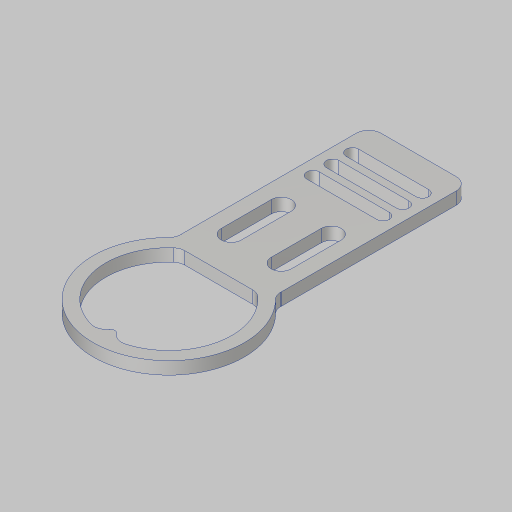
# Autodesk Inventor part: EL2-C-006
Saved by Autodesk Inventor 2023.5 (Build 275446000, 446)
## iProperties
Created: 2025-01-21
Part Number: EL2-C-006
Material: Aluminum 6061
Document SubType Name: Modeling
Designer: slick
Density: 2.7 g/cm^3
Appearance: Aluminum - Flat
Author: slick
Autodesk Inventor part; units mm, degrees
ref_plane "YZ Plane" through (0, 0, 0) normal (1, 0, 0) x (0, 1, 0)
ref_plane "XZ Plane" through (0, 0, 0) normal (0, 1, 0) x (-1, 0, 0)
ref_plane "XY Plane" through (0, 0, 0) normal (0, 0, 1) x (1, 0, 0)
sketch "Sketch1" plane through (0, 0, 0) normal (0, 1, 0) x (-1, 0, 0)
  line L0 (8.89, 0) -> (-8.89, 0) construction
  line L1 (8.89, 1.5875) -> (-8.89, 1.5875)
  line L2 (-8.89, -1.5875) -> (8.89, -1.5875)
  arc A0 (8.89, -1.5875) -> (8.89, 1.5875) centre (8.89, 0) ccw
  arc A1 (-8.89, 1.5875) -> (-8.89, -1.5875) centre (-8.89, 0) ccw
  line L3 (8.89, -5.0038) -> (-8.89, -5.0038) construction
  line L4 (8.89, -3.4163) -> (-8.89, -3.4163)
  line L5 (-8.89, -6.5913) -> (8.89, -6.5913)
  arc A2 (8.89, -6.5913) -> (8.89, -3.4163) centre (8.89, -5.0038) ccw
  arc A3 (-8.89, -3.4163) -> (-8.89, -6.5913) centre (-8.89, -5.0038) ccw
  line L6 (8.89, -10.0076) -> (-8.89, -10.0076) construction
  line L7 (8.89, -8.4201) -> (-8.89, -8.4201)
  line L8 (-8.89, -11.5951) -> (8.89, -11.5951)
  arc A4 (8.89, -11.5951) -> (8.89, -8.4201) centre (8.89, -10.0076) ccw
  arc A5 (-8.89, -8.4201) -> (-8.89, -11.5951) centre (-8.89, -10.0076) ccw
  line L9 (12.7, 32.8549) -> (-12.7, 32.8549)
  line L10 (-12.7, 32.8549) -> (-12.7, -17.9451)
  line L11 (-12.7, -17.9451) -> (12.7, -17.9451)
  line L12 (12.7, -17.9451) -> (12.7, 32.8549)
  line L13 (6.35, 26.5049) -> (-6.35, 26.5049) construction
  point P0 (0, 0)
  point P1 (0, -5.0038)
  point P2 (0, -10.0076)
  point P3 (10.4775, -5.0038)
  point P4 (10.4775, 0)
  point P5 (10.4775, -10.0076)
  point P6 (0, -17.9451)
  point P7 (0, -11.5951)
  point P8 (0, 26.5049)
  point P9 (0, 32.8549)
  dimension "d1" = 17.78
  dimension "d3" = 3.175
  dimension "d4" = 5.0038
  dimension "d5" = 5.0038
  dimension "d8" = 25.4
  dimension "d9" = 50.8
  dimension "d10" = 6.35
  dimension "d11" = 12.7
  dimension "d12" = 6.35
  constraints: 34 end point, 15 point on circle, 12 tangent, 9 parallel, 7 midpoint, 6 centre point, 4 vertical alignment, 3 horizontal, 2 equal radius, 1 horizontal alignment, 1 perpendicular
  measures "d1" distance of L1.start L1.end
  measures "d3" distance between parallel lines of L2 L1
  measures "d4" distance of point (10.477, -5.004) point (10.477, 0)
  measures "d5" distance of point (10.477, -10.008) point (10.477, -5.004)
  measures "d8" distance of L10.end L11.end
  measures "d9" distance of L11.end L9.start
  measures "d10" distance of point (0, -11.595) point (0, -17.945)
  measures "d11" distance of L13.start L13.end
  measures "d12" distance from line of L9 L13.start
extrude "Extrusion1" add sketch "Sketch1" along normal blind 3.175
fillet "Fillet1" radius 3.175 4 edges at (-12.7, 1.5875, -17.9451) (12.7, 1.5875, -17.9451) (12.7, 1.5875, 32.8549) (-12.7, 1.5875, 32.8549)
sketch "Sketch2" plane through (0, 3.175, 0) normal (0, 1, 0) x (1, 0, 0)
  line L0 (-6.35, -10.6299) -> (-6.35, -23.3299) construction
  line L1 (-8.9027, -10.6299) -> (-8.9027, -23.3299)
  line L2 (-3.7973, -23.3299) -> (-3.7973, -10.6299)
  arc A0 (-3.7973, -10.6299) -> (-8.9027, -10.6299) centre (-6.35, -10.6299) ccw
  arc A1 (-8.9027, -23.3299) -> (-3.7973, -23.3299) centre (-6.35, -23.3299) ccw
  line L3 (6.35, -10.6299) -> (6.35, -23.3299) construction
  line L4 (3.7973, -10.6299) -> (3.7973, -23.3299)
  line L5 (8.9027, -23.3299) -> (8.9027, -10.6299)
  arc A2 (8.9027, -10.6299) -> (3.7973, -10.6299) centre (6.35, -10.6299) ccw
  arc A3 (3.7973, -23.3299) -> (8.9027, -23.3299) centre (6.35, -23.3299) ccw
  line L6 (-9.525, -32.8549) -> (9.525, -32.8549) projected
  line L7 (9.525, 17.9451) -> (-9.525, 17.9451) projected
  line L8 (-6.35, -16.9799) -> (6.35, -16.9799) construction
  point P0 (0, 0)
  point P1 (0, -16.9799)
  point P2 (0, 17.9451)
  dimension "d23" = 5.1054
  dimension "d24" = 12.7
  dimension "d26" = 34.925
  dimension "d27" = 12.7
  constraints: 18 end point, 8 point on circle, 8 tangent, 4 centre point, 4 midpoint, 3 parallel, 2 horizontal alignment, 1 equal radius, 1 perpendicular, 1 vertical, 1 vertical alignment
  measures "d23" diameter of A1
  measures "d24" distance of L0.start L0.end
  measures "d26" distance from line of L8.start L7
  measures "d27" distance of L8.start L8.end
extrude "Extrusion2" cut sketch "Sketch2" against normal blind 25.4
sketch "Sketch3" plane through (0, 3.175, 0) normal (0, 1, 0) x (1, 0, 0)
  circle A0 centre (0, -45.5549) radius 16.002
  line L0 (-9.525, -32.8549) -> (9.525, -32.8549) projected
  circle A1 centre (0, -45.5549) radius 19.177
  line L1 (3.7973, -10.6299) -> (3.7973, -23.3299) projected
  arc A2 (3.7973, -23.3299) -> (8.9027, -23.3299) centre (6.35, -23.3299) ccw projected
  line L2 (8.9027, -23.3299) -> (8.9027, -10.6299) projected
  arc A3 (8.9027, -10.6299) -> (3.7973, -10.6299) centre (6.35, -10.6299) ccw projected
  line L3 (-8.9027, -10.6299) -> (-8.9027, -23.3299) projected
  arc A4 (-8.9027, -23.3299) -> (-3.7973, -23.3299) centre (-6.35, -23.3299) ccw projected
  line L4 (-3.7973, -23.3299) -> (-3.7973, -10.6299) projected
  arc A5 (-3.7973, -10.6299) -> (-8.9027, -10.6299) centre (-6.35, -10.6299) ccw projected
  arc A6 (-12.7, -29.6799) -> (-9.525, -32.8549) centre (-9.525, -29.6799) ccw projected
  line L5 (-12.7, -29.6799) -> (-12.7, 14.7701) projected
  arc A7 (-9.525, 17.9451) -> (-12.7, 14.7701) centre (-9.525, 14.7701) ccw projected
  line L6 (-9.525, 17.9451) -> (9.525, 17.9451) projected
  arc A8 (12.7, 14.7701) -> (9.525, 17.9451) centre (9.525, 14.7701) ccw projected
  line L7 (12.7, 14.7701) -> (12.7, -29.6799) projected
  arc A9 (9.525, -32.8549) -> (12.7, -29.6799) centre (9.525, -29.6799) ccw projected
  line L8 (9.525, -32.8549) -> (-9.525, -32.8549) projected
  line L9 (-8.89, -1.5875) -> (8.89, -1.5875) projected
  arc A10 (8.89, -1.5875) -> (8.89, 1.5875) centre (8.89, 0) ccw projected
  line L10 (8.89, 1.5875) -> (-8.89, 1.5875) projected
  arc A11 (-8.89, 1.5875) -> (-8.89, -1.5875) centre (-8.89, 0) ccw projected
  line L11 (-8.89, 3.4163) -> (8.89, 3.4163) projected
  arc A12 (8.89, 3.4163) -> (8.89, 6.5913) centre (8.89, 5.0038) ccw projected
  line L12 (8.89, 6.5913) -> (-8.89, 6.5913) projected
  arc A13 (-8.89, 6.5913) -> (-8.89, 3.4163) centre (-8.89, 5.0038) ccw projected
  line L13 (-8.89, 8.4201) -> (8.89, 8.4201) projected
  arc A14 (8.89, 8.4201) -> (8.89, 11.5951) centre (8.89, 10.0076) ccw projected
  line L14 (8.89, 11.5951) -> (-8.89, 11.5951) projected
  arc A15 (-8.89, 11.5951) -> (-8.89, 8.4201) centre (-8.89, 10.0076) ccw projected
  line L15 (3.7973, -10.6299) -> (3.7973, -23.3299) projected
  arc A16 (3.7973, -23.3299) -> (8.9027, -23.3299) centre (6.35, -23.3299) ccw projected
  line L16 (8.9027, -23.3299) -> (8.9027, -10.6299) projected
  arc A17 (8.9027, -10.6299) -> (3.7973, -10.6299) centre (6.35, -10.6299) ccw projected
  line L17 (-8.9027, -10.6299) -> (-8.9027, -23.3299) projected
  arc A18 (-8.9027, -23.3299) -> (-3.7973, -23.3299) centre (-6.35, -23.3299) ccw projected
  line L18 (-3.7973, -23.3299) -> (-3.7973, -10.6299) projected
  arc A19 (-3.7973, -10.6299) -> (-8.9027, -10.6299) centre (-6.35, -10.6299) ccw projected
  arc A20 (-12.7, -29.6799) -> (-9.525, -32.8549) centre (-9.525, -29.6799) ccw projected
  line L19 (-12.7, -29.6799) -> (-12.7, 14.7701) projected
  arc A21 (-9.525, 17.9451) -> (-12.7, 14.7701) centre (-9.525, 14.7701) ccw projected
  line L20 (-9.525, 17.9451) -> (9.525, 17.9451) projected
  arc A22 (12.7, 14.7701) -> (9.525, 17.9451) centre (9.525, 14.7701) ccw projected
  line L21 (12.7, 14.7701) -> (12.7, -29.6799) projected
  arc A23 (9.525, -32.8549) -> (12.7, -29.6799) centre (9.525, -29.6799) ccw projected
  line L22 (9.525, -32.8549) -> (-9.525, -32.8549) projected
  line L23 (-8.89, -1.5875) -> (8.89, -1.5875) projected
  arc A24 (8.89, -1.5875) -> (8.89, 1.5875) centre (8.89, 0) ccw projected
  line L24 (8.89, 1.5875) -> (-8.89, 1.5875) projected
  arc A25 (-8.89, 1.5875) -> (-8.89, -1.5875) centre (-8.89, 0) ccw projected
  line L25 (-8.89, 3.4163) -> (8.89, 3.4163) projected
  arc A26 (8.89, 3.4163) -> (8.89, 6.5913) centre (8.89, 5.0038) ccw projected
  line L26 (8.89, 6.5913) -> (-8.89, 6.5913) projected
  arc A27 (-8.89, 6.5913) -> (-8.89, 3.4163) centre (-8.89, 5.0038) ccw projected
  line L27 (-8.89, 8.4201) -> (8.89, 8.4201) projected
  arc A28 (8.89, 8.4201) -> (8.89, 11.5951) centre (8.89, 10.0076) ccw projected
  line L28 (8.89, 11.5951) -> (-8.89, 11.5951) projected
  arc A29 (-8.89, 11.5951) -> (-8.89, 8.4201) centre (-8.89, 10.0076) ccw projected
  point P0 (0, 0)
  point P1 (0, -32.8549)
  point P2 (12.433, -30.9543)
  point P3 (9.7268, -32.8485)
  point P4 (-9.7268, -32.8485)
  point P5 (-12.433, -30.9543)
  dimension "d30" = 32.004
  dimension "d31" = 12.7
  dimension "d32" = 3.175
  constraints: 2 centre point, 1 midpoint, 1 vertical alignment
  measures "d30" diameter of A0
  measures "d31" distance from line of L0 A0.centre
  measures "d32" radial gap between concentric circles of A0 A1
extrude "Extrusion3" add sketch "Sketch3" against normal up to surface (3.175 mm away) contours A0 A9 A1 A6 picked at (17.9419, -47.0477)
fillet "Fillet2" radius 3.175 4 edges at (-12.433, 1.5875, 30.9543) (12.433, 1.5875, 30.9543) (9.7268, 1.5875, 32.8485) (-9.7268, 1.5875, 32.8485)
sketch "Sketch4" plane through (0, 3.175, 0) normal (0, 1, 0) x (1, 0, 0)
  circle A0 centre (0, -60.4901) radius 1.1811
  arc A1 (-8.5911, -32.8549) -> (-10.7176, -33.6722) centre (-8.5911, -36.0299) ccw projected
  arc A2 (-10.7176, -33.6722) -> (10.7176, -33.6722) centre (0, -45.5549) ccw projected
  arc A3 (10.7176, -33.6722) -> (8.5911, -32.8549) centre (8.5911, -36.0299) ccw projected
  line L0 (8.5911, -32.8549) -> (-8.5911, -32.8549) projected
  arc A4 (12.6992, -29.749) -> (13.6187, -32.0535) centre (15.8735, -29.8182) ccw projected
  arc A5 (-13.6187, -32.0535) -> (13.6187, -32.0535) centre (0, -45.5549) ccw projected
  arc A6 (-13.6187, -32.0535) -> (-12.6992, -29.749) centre (-15.8735, -29.8182) ccw projected
  arc A7 (-12.7, -29.6799) -> (-12.6992, -29.749) centre (-9.525, -29.6799) ccw projected
  line L1 (-12.7, -29.6799) -> (-12.7, 14.7701) projected
  arc A8 (-9.525, 17.9451) -> (-12.7, 14.7701) centre (-9.525, 14.7701) ccw projected
  line L2 (-9.525, 17.9451) -> (9.525, 17.9451) projected
  arc A9 (12.7, 14.7701) -> (9.525, 17.9451) centre (9.525, 14.7701) ccw projected
  line L3 (12.7, 14.7701) -> (12.7, -29.6799) projected
  arc A10 (12.6992, -29.749) -> (12.7, -29.6799) centre (9.525, -29.6799) ccw projected
  line L4 (3.7973, -10.6299) -> (3.7973, -23.3299) projected
  arc A11 (3.7973, -23.3299) -> (8.9027, -23.3299) centre (6.35, -23.3299) ccw projected
  line L5 (8.9027, -23.3299) -> (8.9027, -10.6299) projected
  arc A12 (8.9027, -10.6299) -> (3.7973, -10.6299) centre (6.35, -10.6299) ccw projected
  line L6 (-8.9027, -10.6299) -> (-8.9027, -23.3299) projected
  arc A13 (-8.9027, -23.3299) -> (-3.7973, -23.3299) centre (-6.35, -23.3299) ccw projected
  line L7 (-3.7973, -23.3299) -> (-3.7973, -10.6299) projected
  arc A14 (-3.7973, -10.6299) -> (-8.9027, -10.6299) centre (-6.35, -10.6299) ccw projected
  line L8 (-8.89, -1.5875) -> (8.89, -1.5875) projected
  arc A15 (8.89, -1.5875) -> (8.89, 1.5875) centre (8.89, 0) ccw projected
  line L9 (8.89, 1.5875) -> (-8.89, 1.5875) projected
  arc A16 (-8.89, 1.5875) -> (-8.89, -1.5875) centre (-8.89, 0) ccw projected
  line L10 (-8.89, 3.4163) -> (8.89, 3.4163) projected
  arc A17 (8.89, 3.4163) -> (8.89, 6.5913) centre (8.89, 5.0038) ccw projected
  line L11 (8.89, 6.5913) -> (-8.89, 6.5913) projected
  arc A18 (-8.89, 6.5913) -> (-8.89, 3.4163) centre (-8.89, 5.0038) ccw projected
  line L12 (-8.89, 8.4201) -> (8.89, 8.4201) projected
  arc A19 (8.89, 8.4201) -> (8.89, 11.5951) centre (8.89, 10.0076) ccw projected
  line L13 (8.89, 11.5951) -> (-8.89, 11.5951) projected
  arc A20 (-8.89, 11.5951) -> (-8.89, 8.4201) centre (-8.89, 10.0076) ccw projected
  point P0 (0, 0)
  point P1 (0, -61.5569)
  point P2 (-0.5246, -61.5483)
  point P3 (0.5246, -61.5483)
  dimension "d36" = 2.3622
  dimension "d37" = 1.0668
  constraints: 1 centre point, 1 point on circle
  measures "d36" diameter of A0
  measures "d37" distance of point (0, -61.557) A0.centre
extrude "Extrusion4" add sketch "Sketch4" against normal up to surface (3.175 mm away) contours A0 A2 picked at (-0.0326, -60.8083)
fillet "Fillet3" radius 3.175 2 edges at (-0.5246, 1.5875, 61.5483) (0.5246, 1.5875, 61.5483)
equation "\"d5\" = d4"
body "Solid1"
